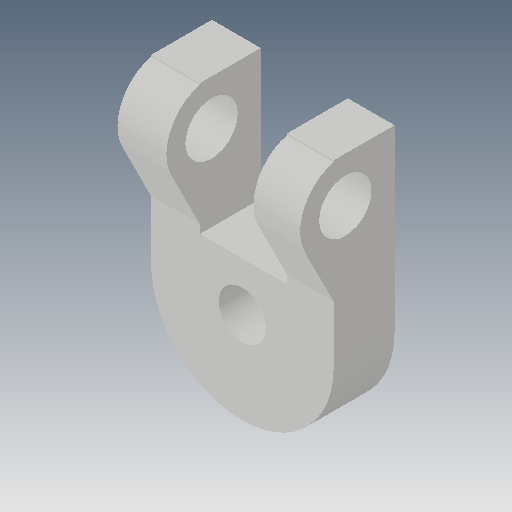
# Autodesk Inventor part: omni wheel short low channel mount
Saved by Autodesk Inventor 2018 (Build 220112000, 112)
## iProperties
Created: 2019-02-06
Part Number: omni wheel short low channel mount
Material: Generic
Document SubType Name: Modeling
Designer: ball
Density: 1 g/cm^3
Appearance: Default
Author: ball
Autodesk Inventor part; units mm, degrees
ref_plane "YZ Plane" through (0, 0, 0) normal (1, 0, 0) x (0, 1, 0)
ref_plane "XZ Plane" through (0, 0, 0) normal (0, 1, 0) x (-1, 0, 0)
sketch "Sketch1" plane through (0, 0, 0) normal (0, 0, 1) x (1, 0, 0)
  arc A0 (-7.62, 0) -> (7.62, 0) centre (0, 0) ccw
  line L0 (1.0603, 17.7117) -> (-0.8757, 17.7117) construction
  line L1 (-7.62, 0) -> (7.62, 0)
  line L2 (7.62, 0) -> (7.62, 14.9733)
  line L3 (7.62, 14.9733) -> (-7.62, 14.9733)
  line L4 (-7.62, 14.9733) -> (-7.62, 0)
  dimension "d0" = 15.24
  dimension "d6" = 14.9733
  constraints: 10 end point, 2 horizontal, 2 parallel, 2 point on circle, 1 centre point, 1 coincident, 1 perpendicular, 2 other
  measures "d0" diameter of A0
  measures "d6" distance between parallel lines of L3 L1
ref_plane "Work Plane1" through (-4.0767, -4.0767, 5.08) normal (0, 0, -1) x (0, 1, 0)
extrude "Extrusion1" add sketch "Sketch1" along normal up to surface (5.08 mm away)
sketch "Sketch2" plane through (7.62, 0, 0) normal (1, 0, 0) x (0, 0, -1)
  circle A0 centre (-4.1045, 11.2117) radius 2 construction
  arc A1 (-0.3326, 11.2117) -> (-7.4701, 9.5087) centre (-4.1045, 11.2117) ccw
  circle A2 centre (-4.1045, 11.2117) radius 6.5 construction
  line L0 (-5.08, 0) -> (-5.08, 14.9733) projected
  line L1 (-5.08, 4.7853) -> (-7.4701, 9.5087)
  line L2 (-5.08, 4.7853) -> (-0.3326, 4.7853)
  line L3 (-0.3326, 4.7853) -> (-0.3326, 11.2117)
  point P0 (0, 0)
  dimension "d3" = 7.5438
  constraints: 6 end point, 2 perpendicular, 2 point on circle, 1 centre point, 1 coincident, 1 point on line, 1 tangent, 2 other
  measures "d3" diameter of A1
extrude "Extrusion2" add sketch "Sketch2" against normal up to surface (15.24 mm away)
sketch "Sketch3" plane through (0, 0, 5.08) normal (0, 0, 1) x (1, 0, 0)
  circle A0 centre (0, 0) radius 4.0767 construction
  line L0 (3.0923, 15.6797) -> (3.0923, 6.7437) construction
  line L1 (-2.9077, 6.7437) -> (-2.9077, 15.6797) construction
  line L2 (3.7273, 15.6797) -> (3.7273, 6.7437) construction
  line L3 (-3.5427, 6.7437) -> (-3.5427, 15.6797) construction
  line L4 (7.62, 14.9733) -> (-7.62, 14.9733) projected
  line L5 (0, 4.0767) -> (3.7273, 4.0767)
  line L6 (3.7273, 4.0767) -> (3.7273, 14.9733)
  line L7 (0, 4.0767) -> (-3.5427, 4.0767)
  line L8 (-3.5427, 4.0767) -> (-3.5427, 14.9733)
  line L9 (3.7273, 15.2774) -> (-3.5427, 15.2774)
  line L10 (-3.5427, 14.9733) -> (-3.5427, 15.2774)
  line L11 (3.7273, 14.9733) -> (3.7273, 15.2774)
  dimension "d7" = 0.635
  dimension "d8" = 0.635
  constraints: 18 end point, 6 point on line, 3 perpendicular, 2 collinear, 2 horizontal, 2 parallel, 1 vertical alignment, 1 other
  measures "d7" distance between parallel lines of L0 L2
  measures "d8" distance between parallel lines of L1 L3
extrude "Extrusion3" cut sketch "Sketch3" along normal through all both and the other way through all
sketch "Sketch4" plane through (7.62, 0, 0) normal (1, 0, 0) x (0, 0, -1)
  arc A0 (-5.08, 14.8553) -> (-7.4701, 9.5087) centre (-4.1045, 11.2117) ccw construction
  circle A1 centre (-4.1045, 11.2117) radius 2.1844
  point P0 (0, 0)
  point P1 (-5.08, 7.5681)
  dimension "d11" = 4.3688
  constraints: 1 centre point, 1 coincident
  measures "d11" diameter of A1
extrude "Extrusion4" cut sketch "Sketch4" against normal through all
sketch "Sketch5" plane through (0, 0, 5.08) normal (0, 0, 1) x (1, 0, 0)
  circle A0 centre (0, 0) radius 1.9685
  dimension "d14" = 3.937
  constraints: 1 centre point, 1 coincident
  measures "d14" diameter of A0
extrude "Extrusion5" cut sketch "Sketch5" against normal through all
equation "\"d12\" = d11"
body "Solid1"
